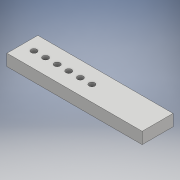
# Autodesk Inventor part: arm
Saved by Autodesk Inventor 2017 (Build 210142000, 142)
## iProperties
Created: 2017-04-18
Part Number: arm
Material: Generic
Document SubType Name: Modeling
Designer: s4461999
Density: 1 g/cm^3
Appearance: Default
Author: s4461999
Autodesk Inventor part; units mm, degrees
ref_plane "YZ Plane" through (0, 0, 0) normal (1, 0, 0) x (0, 1, 0)
ref_plane "XZ Plane" through (0, 0, 0) normal (0, 1, 0) x (-1, 0, 0)
ref_plane "XY Plane" through (0, 0, 0) normal (0, 0, 1) x (1, 0, 0)
sketch "Sketch1" plane through (0, 0, 0) normal (0, 0, 1) x (1, 0, 0)
  line L0 (0, 0) -> (35, 0)
  line L1 (35, 0) -> (35, 8)
  line L2 (35, 8) -> (0, 8)
  line L3 (0, 8) -> (0, 0)
  dimension "d0" = 35
  dimension "d1" = 8
  constraints: 8 end point, 2 parallel, 1 horizontal, 1 perpendicular
  measures "d0" distance of L1.end L2.end
  measures "d1" distance of L0.end L1.end
extrude "Extrusion1" add sketch "Sketch1" along normal blind 3
sketch "Sketch2" plane through (0, 0, 3) normal (0, 0, 1) x (1, 0, 0)
  line L0 (0, 8) -> (0, 0) projected
  line L1 (35, 8) -> (0, 8) projected
  point P0 (3, 4)
  point P1 (6, 4)
  point P2 (9, 4)
  point P3 (12, 4)
  point P4 (15, 4)
  point P5 (18, 4)
  dimension "d4" = 3
  dimension "d5" = 3
  dimension "d6" = 3
  dimension "d7" = 3
  dimension "d8" = 3
  dimension "d9" = 3
  dimension "d10" = 4
  measures "d4" distance from line of point (3, 4) L0
  measures "d5" distance of point (6, 4) point (3, 4)
  measures "d6" distance of point (15, 4) point (18, 4)
  measures "d7" distance of point (12, 4) point (15, 4)
  measures "d8" distance of point (9, 4) point (12, 4)
  measures "d9" distance of point (6, 4) point (9, 4)
  measures "d10" distance from line of L1 point (3, 4)
hole "Hole1" at (3, 4, 3) at (6, 4, 3) at (9, 4, 3) at (12, 4, 3) at (15, 4, 3) at (18, 4, 3) direction (0, 0, -1) diameter 1.5 end through all
body "Solid1"
